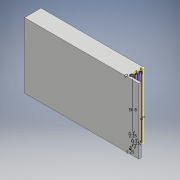
# Autodesk Inventor part: cardBox_attempt1
Saved by Autodesk Inventor 2018 (Build 220112000, 112)
## iProperties
Created: 2019-03-10
Part Number: cardBox_attempt1
Material: Generic
Document SubType Name: Modeling
Designer: natha
Density: 1 g/cm^3
Appearance: Default
Author: natha
Autodesk Inventor part; units mm, degrees
ref_plane "YZ Plane" through (0, 0, 0) normal (1, 0, 0) x (0, 1, 0)
ref_plane "XZ Plane" through (0, 0, 0) normal (0, 1, 0) x (-1, 0, 0)
ref_plane "XY Plane" through (0, 0, 0) normal (0, 0, 1) x (1, 0, 0)
sketch "Sketch1" plane through (0, 0, 0) normal (0, 0, 1) x (1, 0, 0)
  line L0 (-51.45, 7.45) -> (40.55, 7.45)
  line L1 (51.45, -5.45) -> (51.45, -7.45)
  line L2 (51.45, -7.45) -> (-51.45, -7.45)
  line L3 (-51.45, -7.45) -> (-51.45, 7.45)
  line L4 (-51.45, 7.45) -> (51.45, -7.45) construction
  line L5 (51.45, 7.45) -> (-51.45, -7.45) construction
  line L6 (40.55, 7.45) -> (40.55, -5.45)
  line L7 (40.55, -5.45) -> (51.45, -5.45)
  point P0 (0, 0)
  dimension "d0" = 102.9
  dimension "d1" = 14.9
  dimension "d2" = 12.9
  dimension "d3" = 10.9
  constraints: 16 end point, 3 perpendicular, 2 midpoint, 2 parallel, 1 horizontal
  measures "d0" distance of L1.end L2.end
  measures "d1" distance of L5.start L1.end
  measures "d2" distance of L0.end L6.end
  measures "d3" distance between parallel lines of L1 L6
extrude "Extrusion1" add sketch "Sketch1" along normal blind 58.8
sketch "Sketch2" plane through (40.55, -5.45, 0) normal (1, 0, 0) x (0, 0, -1)
  line L0 (0, 0) -> (-58.8, 0) projected
  line L1 (-58.8, 0) -> (-2, 0)
  line L2 (-2, 0) -> (-2, 2.25)
  line L3 (-2, 2.25) -> (-56.8, 2.25)
  line L4 (-58.8, 2.25) -> (-58.8, 0)
  line L5 (0, 12.9) -> (0, 0) projected
  line L6 (-56.8, 2.25) -> (-56.8, 0)
  line L7 (-56.8, 4.8) -> (-2, 4.8)
  line L8 (-2, 4.8) -> (-2, 2.55)
  line L9 (-2, 2.55) -> (-56.8, 2.55)
  line L10 (-58.8, 4.8) -> (-2, 2.55) construction
  line L11 (-2, 4.8) -> (-58.8, 2.55) construction
  line L12 (-56.8, 4.8) -> (-56.8, 2.6292)
  line L13 (-56.8, 5.1) -> (-2, 5.1)
  line L14 (-2, 5.1) -> (-2, 7.35)
  line L15 (-2, 7.35) -> (-56.8, 7.35)
  line L16 (-56.8, 7.35) -> (-56.8, 5.1)
  line L17 (-56.8, 5.1) -> (-2, 7.35) construction
  line L18 (-2, 5.1) -> (-56.8, 7.35) construction
  line L19 (-58.8, 0) -> (-58.8, 12.9) projected
  line L20 (-56.8, 10.9) -> (-2, 10.9)
  line L21 (-2, 10.9) -> (-2, 8.7469)
  line L22 (-2, 8.7469) -> (-56.8, 8.7469)
  line L23 (-56.8, 8.7469) -> (-56.8, 10.9)
  line L24 (-56.8, 10.9) -> (-2, 8.7469) construction
  line L25 (-2, 10.9) -> (-56.8, 8.7469) construction
  line L26 (0, 12.9) -> (-58.8, 12.9) projected
  point P0 (0, 5.45)
  point P1 (-30.4, 3.675)
  point P2 (-29.4, 6.225)
  point P3 (-29.4, 9.8235)
  dimension "d6" = 56.8
  dimension "d7" = 2.25
  dimension "d8" = 2
  dimension "d9" = 2.25
  dimension "d10" = 2
  dimension "d11" = 0.3
  dimension "d12" = 2.25
  dimension "d13" = 2
  dimension "d14" = 0.3
  dimension "d15" = 2.25
  dimension "d16" = 2
  dimension "d17" = 2
  dimension "d18" = 2
  dimension "d19" = 2
  dimension "d20" = 2.25
  constraints: 46 end point, 7 parallel, 6 midpoint, 6 perpendicular, 5 point on line, 3 horizontal
  measures "d6" distance of L1.start L1.end
  measures "d7" distance of L2.end L1.end
  measures "d8" distance between parallel lines of L5 L2
  measures "d9" distance of L4.start L1.start
  measures "d10" distance between parallel lines of L4 L6
  measures "d11" distance between parallel lines of L3 L9
  measures "d12" distance between parallel lines of L9 L7
  measures "d13" distance between parallel lines of L5 L14
  measures "d14" distance between parallel lines of L7 L13
  measures "d15" distance between parallel lines of L15 L13
  measures "d16" distance between parallel lines of L19 L16
  measures "d17" distance between parallel lines of L26 L20
  measures "d18" distance from line of L19 L20.start
  measures "d19" distance between parallel lines of L5 L21
  measures "d20" angle of L25 L20
body "Solid1"
